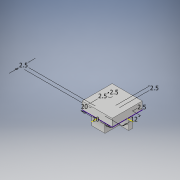
# Autodesk Inventor part: 4
Saved by Autodesk Inventor 2019 (Build 230136000, 136)
## iProperties
Created: 2018-08-09
Part Number: 4
Material: Generic
Document SubType Name: Modeling
Designer: Ge Shi
Density: 1 g/cm^3
Appearance: Default
Author: Ge Shi
Autodesk Inventor part; units mm, degrees
ref_plane "YZ Plane" through (0, 0, 0) normal (1, 0, 0) x (0, 1, 0)
ref_plane "XZ Plane" through (0, 0, 0) normal (0, 1, 0) x (-1, 0, 0)
ref_plane "XY Plane" through (0, 0, 0) normal (0, 0, 1) x (1, 0, 0)
sketch "Sketch1" plane through (0, 0, 0) normal (0, 1, 0) x (-1, 0, 0)
  line L0 (-10, -10) -> (10, -10)
  line L1 (10, -10) -> (10, 10)
  line L2 (10, 10) -> (-10, 10)
  line L3 (-10, 10) -> (-10, -10)
  line L4 (-10, -10) -> (10, 10) construction
  line L5 (10, -10) -> (-10, 10) construction
  line L6 (7.5, 6) -> (7.5, 3.5)
  line L7 (7.5, 3.5) -> (1.25, 3.5)
  line L8 (1.25, 3.5) -> (1.25, -3.5)
  line L9 (1.25, -3.5) -> (7.5, -3.5)
  line L10 (7.5, -3.5) -> (7.5, -6)
  line L11 (7.5, -6) -> (-7.5, -6)
  line L12 (-7.5, -6) -> (-7.5, -3.5)
  line L13 (-7.5, -3.5) -> (-1.25, -3.5)
  line L14 (-1.25, -3.5) -> (-1.25, 6)
  line L15 (-1.25, 6) -> (7.5, 6)
  line L16 (14, 0) -> (-14, 0) projected
  line L17 (0, -14) -> (0, 14) projected
  point P0 (0, 0)
  dimension "d0" = 20
  dimension "d1" = 20
  dimension "d2" = 2.5
  dimension "d3" = 2.5
  dimension "d4" = 12
  dimension "d5" = 2.5
  dimension "d6" = 2.5
  dimension "d7" = 2.5
  constraints: 32 end point, 7 perpendicular, 3 parallel, 2 midpoint, 2 point on line, 1 collinear, 1 horizontal, 1 vertical, 2 other
  measures "d0" distance of L2.end L1.end
  measures "d1" distance of L0.end L1.end
  measures "d2" distance between parallel lines of L1 L10
  measures "d3" distance between parallel lines of L3 L12
  measures "d4" distance from line of L11 L14.end
  measures "d5" distance between parallel lines of L15 L7
  measures "d6" distance of L9.end L10.end
  measures "d7" distance between parallel lines of L14 L8
extrude "Extrusion1" add sketch "Sketch1" against normal blind 10 contours L17 L16 L8 L9 L10 L11 | L11 L12 L13 L14 L16 L17 | L14 L15 L17 L16 | L17 L15 L6 L7 L8 L16
extrude "Extrusion2" add sketch "Sketch1" along normal blind 5
body "Solid1"
